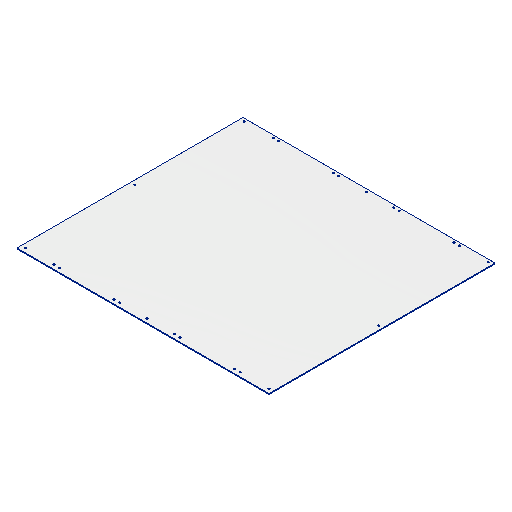
# Autodesk Inventor part: Chapa Base (Trilho Roletado)
Saved by Autodesk Inventor 2026.1 (Build 301233000, 233)
## iProperties
Company: Elgin
Created: 2025-09-16
Part Number: Chapa Base (Trilho Roletado)
Checked By: Antonio Lucas
Engr Approved By: Antonio Lucas
Material: ACM WT SN
Document SubType Name: Modeling
Mfg Approved By: Anderson Oliveira
Designer: Willian Pinheiro
Mass: 6141.43 g
Surface Area: 15283.4 cm^2
Volume: 2274.6 cm^3
Density: 2.7 g/cm^3
Appearance: Alumínio - Plano(1)
Description: Chapa Base (Trilho Roletado)
Dimensões: 3 x 825 x 920 mm
Total: 2
Author: Willian Pinheiro
Title: Ceteva
Revision Number: 00
Autodesk Inventor part; units mm, degrees
ref_plane "YZ Plane" through (0, 0, 0) normal (1, 0, 0) x (0, 1, 0)
ref_plane "XZ Plane" through (0, 0, 0) normal (0, 1, 0) x (-1, 0, 0)
ref_plane "XY Plane" through (0, 0, 0) normal (0, 0, 1) x (1, 0, 0)
sketch "Esboço1" plane through (0, 0, 0) normal (0, 0, 1) x (1, 0, 0)
  line L0 (-644, 0) -> (644, 0) construction
  line L1 (0, -581) -> (0, 581) construction
  line L2 (-460, 415) -> (460, 415)
  line L3 (460, 415) -> (460, -415)
  line L4 (460, -415) -> (-460, -415)
  line L5 (-460, -415) -> (-460, 415)
  line L6 (-445, 415) -> (-445, -415) construction
  line L7 (445, 415) -> (445, -415) construction
  line L8 (-460, -400) -> (460, -400) construction
  line L9 (-460, 400) -> (460, 400) construction
  line L10 (-415, 415) -> (-415, -415) construction
  line L11 (415, 415) -> (415, -415) construction
  line L12 (330, -400) -> (330, 0) construction
  line L13 (220, -400) -> (220, 0) construction
  line L14 (110, -400) -> (110, 0) construction
  line L15 (-330, -400) -> (-330, 0) construction
  line L16 (-110, -400) -> (-110, 0) construction
  point P0 (0, 0)
  point P1 (-445, -400)
  point P2 (-445, 400)
  point P3 (-445, 0)
  point P4 (0, 400)
  point P5 (445, 400)
  point P6 (445, 0)
  point P7 (0, -400)
  point P8 (445, -400)
  point P9 (340, -400)
  point P10 (320, -400)
  point P11 (100, -400)
  point P12 (120, -400)
  point P13 (-340, -400)
  point P14 (-320, -400)
  point P15 (-220, -400)
  point P16 (-120, -400)
  point P17 (-100, -400)
  point P18 (340, 400)
  point P19 (320, 400)
  point P20 (120, 400)
  point P21 (100, 400)
  point P22 (-330, 400)
  point P23 (-100, 400)
  point P24 (-120, 400)
  point P25 (-320, 400)
  point P26 (-340, 400)
  dimension "d0" = 920
  dimension "d1" = 830
  dimension "d2" = 15
  dimension "d3" = 30
  dimension "d4" = 15
  dimension "d20" = 220
  dimension "d21" = 20
  dimension "d22" = 220
  constraints: 30 end point, 29 symmetric about line, 20 point on line, 7 perpendicular, 2 midpoint, 2 parallel, 1 horizontal, 1 vertical, 4 other
  measures "d0" distance of L2.start L2.end
  measures "d1" distance of L4.end L2.start
  measures "d2" distance between parallel lines of L5 L6
  measures "d3" distance between parallel lines of L10 L6
  measures "d4" distance between parallel lines of L2 L9
  measures "d20" distance between parallel lines of L12 L14
  measures "d21" distance of point (340, -400) point (320, -400)
  measures "d22" distance between parallel lines of L14 L16
extrude "Extrusão1" add sketch "Esboço1" against normal blind 3
hole "Furo1" at (-445, -400, 0) at (-445, 400, 0) at (-445, 0, 0) at (0, 400, 0) at (445, 0, 0) at (445, 400, 0) at (0, -400, 0) at (445, -400, 0) direction (0, 0, -1) diameter 6.5 end through all clearance for "Countersunk Flat Head Hex Socket Screw ISO 10642" size "M6" standard "ISO"
hole "Furo2" at (340, -400, 0) at (320, -400, 0) at (120, -400, 0) at (100, -400, 0) at (-100, -400, 0) at (-120, -400, 0) at (-320, -400, 0) at (-340, -400, 0) at (-340, 400, 0) at (-320, 400, 0) at (-120, 400, 0) at (-100, 400, 0) at (100, 400, 0) at (120, 400, 0) at (320, 400, 0) at (340, 400, 0) direction (0, 0, -1) diameter 6.5 end through all clearance for "Countersunk Flat Head Hex Socket Screw ISO 10642" size "M6" standard "ISO"
chamfer "Chanfro1" distance 1 angle 45 4 edges at (-460, -415, -1.5) (-460, 415, -1.5) (460, 415, -1.5) (460, -415, -1.5)
move faces "Mover1" translate (0, -5, 0) faces at (153, 415, -1) (459.3333, 414.6667, -1) (-459.6667, 414.3333, -1)
equation "\"d22\" = d20"
